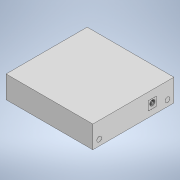
# Autodesk Inventor part: NETGEAR GS305
Saved by Autodesk Inventor 2020.2 (Build 242310000, 310)
## iProperties
Created: 2020-02-15
Part Number: NETGEAR GS305
Material: Generic
Document SubType Name: Modeling
Designer: mulve
Density: 1 g/cm^3
Appearance: Default
Author: mulve
Autodesk Inventor part; units mm, degrees
ref_plane "YZ Plane" through (0, 0, 0) normal (1, 0, 0) x (0, 1, 0)
ref_plane "XZ Plane" through (0, 0, 0) normal (0, 1, 0) x (-1, 0, 0)
ref_plane "XY Plane" through (0, 0, 0) normal (0, 0, 1) x (1, 0, 0)
sketch "Sketch1" plane through (0, 0, 0) normal (0, 1, 0) x (-1, 0, 0)
  line L0 (0, 0) -> (100.79, 0)
  line L1 (100.79, 0) -> (100.79, -94.25)
  line L2 (100.79, -94.25) -> (0, -94.25)
  line L3 (0, -94.25) -> (0, 0)
  dimension "d0" = 94.25
  dimension "d1" = 100.79
  constraints: 8 end point, 2 parallel, 1 horizontal, 1 perpendicular
  measures "d0" distance of L0.end L1.end
  measures "d1" distance of L1.end L2.end
extrude "Extrusion1" add sketch "Sketch1" along normal blind 25.9
sketch "Sketch2" plane through (0, 0, 0) normal (1, 0, 0) x (0, 0, -1)
  circle A0 centre (7.5, 6.9) radius 2.8
  circle A1 centre (86.75, 6.9) radius 2.8
  line L0 (0, 25.9) -> (94.25, 25.9) projected
  line L1 (94.25, 0) -> (94.25, 25.9) projected
  line L2 (0, 0) -> (0, 25.9) projected
  dimension "d4" = 5.6
  dimension "d5" = 19
  dimension "d6" = 19
  dimension "d7" = 7.5
  dimension "d8" = 7.5
  constraints: 2 centre point, 1 equal radius
  measures "d4" diameter of A1
  measures "d5" distance from line of L0 A1.centre
  measures "d6" distance from line of L0 A0.centre
  measures "d7" distance from line of L1 A1.centre
  measures "d8" distance from line of L2 A0.centre
extrude "Extrusion2" cut sketch "Sketch2" against normal blind 0.1
sketch "Sketch3" plane through (0, 0, 0) normal (1, 0, 0) x (0, 0, -1)
  line L0 (64.5, 17.04) -> (73.93, 17.04)
  line L1 (73.93, 17.04) -> (73.93, 6.7)
  line L2 (73.93, 6.7) -> (64.5, 6.7)
  line L3 (64.5, 6.7) -> (64.5, 17.04)
  line L4 (0, 0) -> (94.25, 0) projected
  line L5 (0, 25.9) -> (94.25, 25.9) projected
  line L6 (94.25, 0) -> (94.25, 25.9) projected
  line L7 (0, 0) -> (0, 25.9) projected
  circle A0 centre (69.215, 12.64) radius 3.05
  circle A1 centre (69.215, 12.64) radius 1.2
  dimension "d11" = 6.7
  dimension "d12" = 8.86
  dimension "d13" = 20.32
  dimension "d14" = 64.5
  dimension "d15" = 6.1
  dimension "d16" = 2.4
  dimension "d17" = 4.4
  constraints: 8 end point, 2 centre point, 2 parallel, 1 coincident, 1 horizontal, 1 perpendicular
  measures "d11" distance between parallel lines of L4 L2
  measures "d12" distance between parallel lines of L5 L0
  measures "d13" distance between parallel lines of L6 L1
  measures "d14" distance between parallel lines of L7 L3
  measures "d15" diameter of A0
  measures "d16" diameter of A1
  measures "d17" distance from line of L0 A0.centre
extrude "Extrusion3" cut sketch "Sketch3" against normal blind 10.33 contours A0
extrude "Extrusion4" cut sketch "Sketch3" against normal blind 0.1 contours L0 L1 L2 L3
sketch "Sketch4" plane through (-100.79, 0, -94.25) normal (-1, 0, 0) x (0, 0, 1)
  line L0 (10.48, 18.65) -> (73.15, 18.65)
  line L1 (73.15, 18.65) -> (73.15, 5.73)
  line L2 (73.15, 5.73) -> (10.48, 5.73)
  line L3 (10.48, 5.73) -> (10.48, 18.65)
  line L4 (0, 0) -> (0, 25.9) projected
  line L5 (0, 25.9) -> (94.25, 25.9) projected
  line L6 (0, 0) -> (94.25, 0) projected
  line L7 (73.15, 18.65) -> (88.7, 18.65)
  line L8 (88.7, 18.65) -> (88.7, 5.73)
  line L9 (88.7, 5.73) -> (73.15, 5.73)
  line L10 (73.15, 5.73) -> (73.15, 18.65)
  line L11 (11.98, 7.83) -> (23.98, 7.83)
  line L12 (23.98, 7.83) -> (23.98, 14.59)
  line L13 (23.98, 14.59) -> (11.98, 14.59)
  line L14 (11.98, 14.59) -> (11.98, 7.83)
  line L15 (11.18, 12.61) -> (24.78, 12.61)
  line L16 (24.78, 12.61) -> (24.78, 9.61)
  line L17 (24.78, 9.61) -> (11.18, 9.61)
  line L18 (11.18, 9.61) -> (11.18, 12.61)
  line L19 (14.89, 7.83) -> (21.13, 7.83)
  line L20 (21.13, 7.83) -> (21.13, 16.24)
  line L21 (21.13, 16.24) -> (14.89, 16.24)
  line L22 (14.89, 16.24) -> (14.89, 7.83)
  line L23 (16.01, 7.83) -> (20.01, 7.83)
  line L24 (20.01, 7.83) -> (20.01, 17.48)
  line L25 (20.01, 17.48) -> (16.01, 17.48)
  line L26 (16.01, 17.48) -> (16.01, 7.83)
  line L27 (25.81, 5.73) -> (25.81, 18.65) construction
  line L28 (39.64, 7.83) -> (27.64, 7.83)
  line L29 (27.64, 7.83) -> (27.64, 14.59)
  line L30 (27.64, 14.59) -> (39.64, 14.59)
  line L31 (39.64, 14.59) -> (39.64, 7.83)
  line L32 (40.44, 12.61) -> (26.84, 12.61)
  line L33 (26.84, 12.61) -> (26.84, 9.61)
  line L34 (26.84, 9.61) -> (40.44, 9.61)
  line L35 (40.44, 9.61) -> (40.44, 12.61)
  line L36 (30.49, 7.83) -> (30.49, 16.24)
  line L37 (30.49, 16.24) -> (36.73, 16.24)
  line L38 (36.73, 16.24) -> (36.73, 7.83)
  line L39 (31.61, 7.83) -> (31.61, 17.48)
  line L40 (31.61, 17.48) -> (35.61, 17.48)
  line L41 (35.61, 17.48) -> (35.61, 7.83)
  line L42 (41.47, 5.73) -> (41.47, 18.65) construction
  line L43 (70.96, 7.83) -> (58.96, 7.83)
  line L44 (58.96, 7.83) -> (58.96, 14.59)
  line L45 (58.96, 14.59) -> (70.96, 14.59)
  line L46 (70.96, 14.59) -> (70.96, 7.83)
  line L47 (71.76, 12.61) -> (58.16, 12.61)
  line L48 (58.16, 12.61) -> (58.16, 9.61)
  line L49 (58.16, 9.61) -> (71.76, 9.61)
  line L50 (71.76, 9.61) -> (71.76, 12.61)
  line L51 (61.81, 7.83) -> (61.81, 16.24)
  line L52 (61.81, 16.24) -> (68.05, 16.24)
  line L53 (68.05, 16.24) -> (68.05, 7.83)
  line L54 (62.93, 7.83) -> (62.93, 17.48)
  line L55 (62.93, 17.48) -> (66.93, 17.48)
  line L56 (66.93, 17.48) -> (66.93, 7.83)
  line L57 (51.33, 17.48) -> (47.33, 17.48)
  line L58 (47.33, 17.48) -> (47.33, 7.83)
  line L59 (52.45, 16.24) -> (46.21, 16.24)
  line L60 (46.21, 16.24) -> (46.21, 7.83)
  line L61 (55.3, 14.59) -> (43.3, 14.59)
  line L62 (43.3, 14.59) -> (43.3, 7.83)
  line L63 (42.5, 12.61) -> (56.1, 12.61)
  line L64 (42.5, 9.61) -> (42.5, 12.61)
  line L65 (56.1, 9.61) -> (42.5, 9.61)
  line L66 (43.3, 7.83) -> (55.3, 7.83)
  line L67 (51.33, 7.83) -> (51.33, 17.48)
  line L68 (52.45, 7.83) -> (52.45, 16.24)
  line L69 (55.3, 7.83) -> (55.3, 14.59)
  line L70 (56.1, 12.61) -> (56.1, 9.61)
  line L71 (74.9411, 7.83) -> (74.9411, 14.59)
  line L72 (74.125, 12.61) -> (74.125, 9.61)
  line L73 (77.7911, 7.83) -> (77.7911, 16.24)
  line L74 (78.9111, 7.83) -> (78.9111, 17.48)
  line L75 (74.9411, 14.59) -> (86.9411, 14.59)
  line L76 (87.725, 12.61) -> (74.125, 12.61)
  line L77 (74.125, 9.61) -> (87.725, 9.61)
  line L78 (86.9411, 7.83) -> (74.9411, 7.83)
  line L79 (84.0311, 16.24) -> (84.0311, 7.83)
  line L80 (82.9111, 17.48) -> (82.9111, 7.83)
  line L81 (87.725, 9.61) -> (87.725, 12.61)
  line L82 (86.9411, 14.59) -> (86.9411, 7.83)
  line L83 (77.7911, 16.24) -> (84.0311, 16.24)
  line L84 (78.9111, 17.48) -> (82.9111, 17.48)
  point P0 (16.01, 16.24)
  point P1 (14.89, 14.59)
  point P2 (11.98, 12.61)
  point P3 (11.98, 9.61)
  point P4 (23.98, 9.61)
  point P5 (23.98, 12.61)
  point P6 (21.13, 14.59)
  point P7 (20.01, 16.24)
  point P8 (86.9411, 9.61)
  point P9 (86.9411, 12.61)
  point P10 (84.0311, 14.59)
  point P11 (82.9111, 16.24)
  point P12 (78.9111, 16.24)
  point P13 (77.7911, 14.59)
  point P14 (74.9411, 12.61)
  point P15 (74.9411, 9.61)
  point P16 (58.96, 12.61)
  point P17 (58.96, 9.61)
  point P18 (70.96, 9.61)
  point P19 (70.96, 12.61)
  point P20 (68.05, 14.59)
  point P21 (66.93, 16.24)
  point P22 (62.93, 16.24)
  point P23 (61.81, 14.59)
  point P24 (55.3, 12.61)
  point P25 (52.45, 14.59)
  point P26 (51.33, 16.24)
  point P27 (47.33, 16.24)
  point P28 (46.21, 14.59)
  point P29 (43.3, 12.61)
  point P30 (43.3, 9.61)
  point P31 (55.3, 9.61)
  point P32 (27.64, 12.61)
  point P33 (27.64, 9.61)
  point P34 (39.64, 9.61)
  point P35 (39.64, 12.61)
  point P36 (36.73, 14.59)
  point P37 (35.61, 16.24)
  point P38 (31.61, 16.24)
  point P39 (30.49, 14.59)
  dimension "d22" = 62.67
  dimension "d23" = 10.48
  dimension "d24" = 12.92
  dimension "d27" = 15.55
  dimension "d28" = 12
  dimension "d29" = 6.76
  dimension "d30" = 2.1
  dimension "d31" = 1.5
  dimension "d32" = 13.6
  dimension "d33" = 3
  dimension "d34" = 0.8
  dimension "d35" = 0.8
  dimension "d36" = 3.88
  dimension "d37" = 6.24
  dimension "d38" = 4.41
  dimension "d39" = 8.41
  dimension "d40" = 9.65
  dimension "d41" = 4
  dimension "d42" = 1.12
  dimension "d43" = 1.12
  dimension "d48" = 1.03
  dimension "d49" = 1.03
  dimension "d50" = 0.975
  dimension "d51" = 0.975
  dimension "d58" = 5.73
  dimension "d59" = 12.92
  constraints: 164 end point, 48 symmetric about line, 12 parallel, 10 equal length, 10 point on line, 8 perpendicular, 6 collinear, 6 horizontal
  measures "d22" distance of L1.end L2.end
  measures "d23" distance between parallel lines of L4 L3
  measures "d24" distance of L0.end L1.end
  measures "d27" distance of L0.end L7.end
  measures "d28" distance of L11.start L11.end
  measures "d29" distance of L11.end L12.end
  measures "d30" distance between parallel lines of L2 L11
  measures "d31" distance between parallel lines of L3 L14
  measures "d32" distance of L15.start L15.end
  measures "d33" distance of L15.end L16.end
  measures "d34" distance between parallel lines of L12 L16
  measures "d35" distance between parallel lines of L14 L18
  measures "d36" distance between parallel lines of L2 L17
  measures "d37" distance of L20.end L21.end
  measures "d38" distance between parallel lines of L3 L22
  measures "d39" distance of L19.end L20.end
  measures "d40" distance of L23.end L24.end
  measures "d41" distance of L24.end L25.end
  measures "d42" distance between parallel lines of L22 L26
  measures "d43" distance between parallel lines of L20 L24
  measures "d48" distance between parallel lines of L16 L27
  measures "d49" distance between parallel lines of L35 L42
  measures "d50" distance between parallel lines of L8 L81
  measures "d51" distance between parallel lines of L1 L72
  measures "d58" distance between parallel lines of L6 L2
  measures "d59" distance of L7.end L8.end
extrude "Extrusion5" cut sketch "Sketch4" against normal blind 12.41 contours L14 L17 L22 L11 | L22 L17 L26 L11 | L17 L18 L15 L14 | L14 L15 L22 L17 | L26 L17 L24 L11 | L22 L15 L26 L17 | L14 L13 L22 L15 | L24 L17 L20 L11 | L26 L15 L24 L17 | L22 L13 L26 L15 | L20 L17 L12 L11 | L24 L15 L20 L17 | L26 L13 L24 L15 | L22 L21 L26 L13 | L20 L15 L12 L17 | L24 L13 L20 L15 | L26 L21 L24 L13 | L12 L15 L16 L17 | L20 L13 L12 L15 | L24 L21 L20 L13 | L26 L25 L24 L21
extrude "Extrusion6" cut sketch "Sketch4" against normal blind 0.1 contours L0 L1 L2 L3 | L7 L8 L9 L1 | L28 L38 L34 L31 | L28 L41 L34 L38 | L34 L38 L32 L31 | L31 L32 L35 L34 | L28 L39 L34 L41 | L34 L41 L32 L38 | L32 L38 L30 L31 | L28 L36 L34 L39 | L34 L39 L32 L41 | L32 L41 L30 L38 | L28 L29 L34 L36 | L34 L36 L32 L39 | L32 L39 L30 L41 | L30 L41 L37 L38 | L34 L29 L32 L36 | L32 L36 L30 L39 | L30 L39 L37 L41 | L34 L33 L32 L29 | L32 L29 L30 L36 | L30 L36 L37 L39 | L37 L39 L40 L41 | L43 L53 L49 L46 | L43 L56 L49 L53 | L49 L53 L47 L46 | L46 L47 L50 L49 | L43 L54 L49 L56 | L49 L56 L47 L53 | L47 L53 L45 L46 | L43 L51 L49 L54 | L49 L54 L47 L56 | L47 L56 L45 L53 | L43 L44 L49 L51 | L49 L51 L47 L54 | L47 L54 L45 L56 | L45 L56 L52 L53 | L49 L44 L47 L51 | L47 L51 L45 L54 | L45 L54 L52 L56 | L49 L48 L47 L44 | L47 L44 L45 L51 | L45 L51 L52 L54 | L52 L54 L55 L56 | L67 L59 L58 L57 | L67 L61 L58 L59 | L59 L68 L61 L67 | L58 L61 L60 L59 | L67 L63 L58 L61 | L61 L68 L63 L67 | L58 L63 L60 L61 | L61 L69 L63 L68 | L67 L65 L58 L63 | L63 L68 L65 L67 | L58 L65 L60 L63 | L60 L63 L62 L61 | L63 L69 L65 L68 | L67 L66 L58 L65 | L65 L68 L66 L67 | L58 L66 L60 L65 | L60 L65 L62 L63 | L63 L70 L65 L69 | L65 L69 L66 L68 | L60 L66 L62 L65 | L62 L65 L64 L63 | L71 L77 L73 L78 | L77 L72 L76 L71 | L71 L76 L73 L77 | L73 L77 L74 L78 | L71 L75 L73 L76 | L73 L76 L74 L77 | L74 L77 L80 L78 | L73 L75 L74 L76 | L74 L76 L80 L77 | L80 L77 L79 L78 | L73 L83 L74 L75 | L74 L75 L80 L76 | L80 L76 L79 L77 | L79 L77 L82 L78 | L74 L83 L80 L75 | L80 L75 L79 L76 | L79 L76 L82 L77 | L74 L84 L80 L83 | L80 L83 L79 L75 | L79 L75 L82 L76 | L82 L76 L81 L77
extrude "Extrusion7" cut sketch "Sketch4" against normal blind 12.41 contours L28 L38 L34 L31 | L28 L41 L34 L38 | L34 L38 L32 L31 | L31 L32 L35 L34 | L28 L39 L34 L41 | L34 L41 L32 L38 | L32 L38 L30 L31 | L28 L36 L34 L39 | L34 L39 L32 L41 | L32 L41 L30 L38 | L28 L29 L34 L36 | L34 L36 L32 L39 | L32 L39 L30 L41 | L30 L41 L37 L38 | L34 L29 L32 L36 | L32 L36 L30 L39 | L30 L39 L37 L41 | L34 L33 L32 L29 | L32 L29 L30 L36 | L30 L36 L37 L39 | L37 L39 L40 L41 | L43 L53 L49 L46 | L43 L56 L49 L53 | L49 L53 L47 L46 | L46 L47 L50 L49 | L43 L54 L49 L56 | L49 L56 L47 L53 | L47 L53 L45 L46 | L43 L51 L49 L54 | L49 L54 L47 L56 | L47 L56 L45 L53 | L43 L44 L49 L51 | L49 L51 L47 L54 | L47 L54 L45 L56 | L45 L56 L52 L53 | L49 L44 L47 L51 | L47 L51 L45 L54 | L45 L54 L52 L56 | L49 L48 L47 L44 | L47 L44 L45 L51 | L45 L51 L52 L54 | L52 L54 L55 L56 | L67 L59 L58 L57 | L67 L61 L58 L59 | L59 L68 L61 L67 | L58 L61 L60 L59 | L67 L63 L58 L61 | L61 L68 L63 L67 | L58 L63 L60 L61 | L61 L69 L63 L68 | L67 L65 L58 L63 | L63 L68 L65 L67 | L58 L65 L60 L63 | L60 L63 L62 L61 | L63 L69 L65 L68 | L67 L66 L58 L65 | L65 L68 L66 L67 | L58 L66 L60 L65 | L60 L65 L62 L63 | L63 L70 L65 L69 | L65 L69 L66 L68 | L60 L66 L62 L65 | L62 L65 L64 L63 | L71 L77 L73 L78 | L77 L72 L76 L71 | L71 L76 L73 L77 | L73 L77 L74 L78 | L71 L75 L73 L76 | L73 L76 L74 L77 | L74 L77 L80 L78 | L73 L75 L74 L76 | L74 L76 L80 L77 | L80 L77 L79 L78 | L73 L83 L74 L75 | L74 L75 L80 L76 | L80 L76 L79 L77 | L79 L77 L82 L78 | L74 L83 L80 L75 | L80 L75 L79 L76 | L79 L76 L82 L77 | L74 L84 L80 L83 | L80 L83 L79 L75 | L79 L75 L82 L76 | L82 L76 L81 L77
sketch "Sketch5" plane through (-100.79, 0, -94.25) normal (-1, 0, 0) x (0, 0, 1)
  line L0 (3.31, 5.2) -> (8.31, 5.2)
  line L1 (8.31, 5.2) -> (8.31, 7.6)
  line L2 (8.31, 7.6) -> (3.31, 7.6)
  line L3 (3.31, 7.6) -> (3.31, 5.2)
  line L4 (0, 0) -> (94.25, 0) projected
  line L5 (0, 0) -> (0, 25.9) projected
  dimension "d54" = 5
  dimension "d55" = 2.4
  dimension "d56" = 5.2
  dimension "d57" = 3.31
  constraints: 8 end point, 2 parallel, 1 horizontal, 1 perpendicular
  measures "d54" distance of L0.start L0.end
  measures "d55" distance of L0.end L1.end
  measures "d56" distance between parallel lines of L4 L0
  measures "d57" distance between parallel lines of L5 L3
sketch "Sketch6" plane through (0, 0, 0) normal (0, -1, 0) x (1, 0, 0)
  circle A0 centre (-85.99, -82.59) radius 6.7
  circle A1 centre (-85.99, -11.66) radius 6.7
  circle A2 centre (-20.4, -11.66) radius 6.7
  circle A3 centre (-20.4, -82.59) radius 6.7
  line L0 (-100.79, 0) -> (0, 0) projected
  line L1 (0, -94.25) -> (-100.79, -94.25) projected
  line L2 (-100.79, -94.25) -> (-100.79, 0) projected
  line L3 (0, 0) -> (0, -94.25) projected
  dimension "d60" = 13.4
  dimension "d61" = 11.66
  dimension "d62" = 11.66
  dimension "d63" = 11.66
  dimension "d64" = 11.66
  dimension "d65" = 14.8
  dimension "d66" = 14.8
  dimension "d67" = 20.4
  dimension "d68" = 20.4
  constraints: 4 centre point, 3 equal radius
  measures "d60" diameter of A0
  measures "d61" distance from line of L0 A1.centre
  measures "d62" distance from line of L0 A2.centre
  measures "d63" distance from line of L1 A3.centre
  measures "d64" distance from line of L1 A0.centre
  measures "d65" distance from line of L2 A1.centre
  measures "d66" distance from line of L2 A0.centre
  measures "d67" distance from line of L3 A2.centre
  measures "d68" distance from line of L3 A3.centre
extrude "Extrusion8" cut sketch "Sketch6" against normal blind 0.5 contours A0 | A1 | A2 | A3
sketch "Sketch8" plane through (-85.99, 0.5, -82.59) normal (0, -1, 0) x (1, 0, 0)
  circle A0 centre (0, 0) radius 6
  line L0 (0, 0) -> (0, 71.3591)
  line L1 (0, 0) -> (66.0245, 0)
  circle A1 centre (0, 71) radius 6
  circle A2 centre (65.5, 0) radius 6
  circle A3 centre (65.5, 71) radius 6
  point P0 (85.99, 82.59)
  dimension "d71" = 12
  dimension "d74" = 71
  dimension "d77" = 65.5
  constraints: 4 centre point, 4 end point, 2 horizontal, 2 vertical, 6 other
  measures "d71" diameter of A0
  measures "d74" distance of L0.start A1.centre
  measures "d77" distance of L0.start A2.centre
extrude "Extrusion9" add sketch "Sketch8" along normal blind 1
sketch "Sketch9" plane through (-85.99, -0.5, -82.59) normal (0, -1, 0) x (1, 0, 0)
  circle A0 centre (0, 0) radius 4.625
  line L0 (0, 0) -> (0, 72.6504)
  line L1 (0, 0) -> (66.3076, 0)
  circle A1 centre (0, 71) radius 4.625
  circle A2 centre (65.5, 0) radius 4.625
  circle A3 centre (65.5, 71) radius 4.625
  point P0 (85.99, 82.59)
  dimension "d82" = 9.25
  dimension "d85" = 71
  dimension "d88" = 65.5
  constraints: 4 centre point, 4 end point, 2 horizontal, 2 vertical, 6 other
  measures "d82" diameter of A0
  measures "d85" distance of L0.start A1.centre
  measures "d88" distance of L0.start A2.centre
extrude "Extrusion10" add sketch "Sketch9" along normal blind 2.64
extrude "Extrusion11" cut sketch "Sketch5" against normal blind 0.1
equation "\"d6\" = d5"
equation "\"d8\" = d7"
equation "\"d34\" = d35"
equation "\"d42\" = d43"
equation "\"d49\" = d48"
equation "\"d50\" = d51"
equation "\"d59\" = d24"
equation "\"d62\" = d61"
equation "\"d63\" = d62"
equation "\"d64\" = d61"
equation "\"d66\" = d65"
equation "\"d68\" = d67"
body "Solid1"
